# Autodesk Inventor part: LP2985-33DBVT
Saved by Autodesk Inventor 2016 (Build 200138000, 138)
## iProperties
Created: 2016-04-08
Part Number: LP2985-33DBVT
Material: Generic
Document SubType Name: Modeling
Designer: Paschalis
Density: 1 g/cm^3
Appearance: SOT95P280X145-5N, LP2985-33DBVT
Author: Paschalis
Autodesk Inventor part; units mm, degrees
ref_plane "YZ Plane" through (0, 0, 0) normal (1, 0, 0) x (0, 1, 0)
ref_plane "XZ Plane" through (0, 0, 0) normal (0, 1, 0) x (-1, 0, 0)
ref_plane "XY Plane" through (0, 0, 0) normal (0, 0, 1) x (1, 0, 0)
sketch "SOT95P280X145-5N, LP2985-33DBVT_79" plane through (0, 0, 0) normal (0, 0, 1) x (1, 0, 0)
  line L0 (-1.4986, 1.524) -> (1.4986, 1.524)
  line L1 (1.4986, 1.524) -> (1.4986, -1.6002)
  line L2 (1.4986, -1.6002) -> (-1.4986, -1.6002)
  line L3 (-1.4986, -1.6002) -> (-1.4986, 1.524)
  constraints: 8 end point
extrude "Extrusion1" add sketch "SOT95P280X145-5N, LP2985-33DBVT_79" along normal blind 1
body "Solid1"
